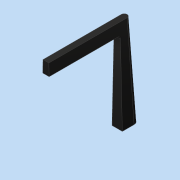
# Autodesk Inventor part: RudderStabilizingFins
Saved by Autodesk Inventor 2017 (Build 210142000, 142)
## iProperties
Created: 2016-10-10
Part Number: RudderStabilizingFins
Material: Generic
Document SubType Name: Modeling
Designer: techn
Density: 1 g/cm^3
Appearance: Glossy - Black
Author: techn
Autodesk Inventor part; units mm, degrees
ref_plane "YZ Plane" through (0, 0, 0) normal (1, 0, 0) x (0, 1, 0)
ref_plane "XY Plane" through (0, 0, 0) normal (0, 0, 1) x (1, 0, 0)
sketch "Sketch6" plane through (0, 0, 0) normal (0, 1, 0) x (-1, 0, 0)
  line L0 (0, 0) -> (5.588, 0)
  line L1 (5.588, 0) -> (5.588, -6.35)
  line L2 (5.588, -6.35) -> (0, -6.35)
  line L3 (0, -6.35) -> (0, 0)
  arc A0 (0, -6.35) -> (5.588, -6.35) centre (2.794, -6.35) ccw
  dimension "d25" = 5.588
  dimension "d26" = 6.35
  constraints: 8 end point, 2 parallel, 2 point on circle, 2 tangent, 1 centre point, 1 horizontal, 1 perpendicular
  measures "d25" distance of L1.end L2.end
  measures "d26" distance of L0.end L1.end
ref_plane "Work Plane1" through (0, 50.8, 0) normal (0, 1, 0) x (-1, 0, 0)
sketch "Sketch8" plane through (0, 50.8, 0) normal (0, 1, 0) x (-1, 0, 0)
  line L0 (4.3815, 0) -> (1.2065, 0)
  line L1 (1.2065, 0) -> (1.2065, -3.81)
  line L2 (1.2065, -3.81) -> (4.3815, -3.81)
  line L3 (4.3815, -3.81) -> (4.3815, 0)
  arc A0 (1.2065, -3.81) -> (4.3815, -3.81) centre (2.794, -3.81) ccw
  point P0 (0, 0)
  dimension "d27" = 3.175
  dimension "d28" = 3.81
  dimension "d49" = 1.2065
  constraints: 8 end point, 2 parallel, 2 point on circle, 2 tangent, 1 centre point, 1 horizontal, 1 perpendicular, 1 point on line
  measures "d27" distance of L2.end L1.end
  measures "d28" distance of L1.end L0.end
  measures "d49" distance from line of point (0, 0) L1
loft "Loft1" add profiles "Sketch6", "Sketch8"
sketch "Sketch9" plane through (-5.588, 0, 0) normal (0, 0, 1) x (1, 0, 0)
  line L0 (0, 0) -> (5.588, 0) projected
  line L1 (5.588, 0) -> (4.3815, 50.8) projected
  line L2 (1.2065, 50.8) -> (4.3815, 50.8) projected
  line L3 (0, 0) -> (1.2065, 50.8) projected
  line L4 (4.3815, 50.8) -> (5.588, 0) projected
  line L5 (4.5323, 44.45) -> (1.0557, 44.45)
  line L6 (0, 0) -> (1.2065, 50.8) projected
  dimension "d34" = 6.35
  constraints: 2 end point, 2 point on line, 1 horizontal
  measures "d34" distance between parallel lines of L2 L5
extrude "Extrusion5" add sketch "Sketch9" along normal blind 38.608 contours L3 L2 L1 L5
fillet "Fillet2" radius 1.5875 1 edges at (-2.794, 44.45, 0)
sketch "Sketch12" plane through (-2.794, 0, -6.35) normal (0, -1, 0) x (1, 0, 0)
  circle A0 centre (0, 1.9685) radius 1.27
  arc A1 (-2.794, 0) -> (2.794, 0) centre (0, 0) ccw projected
  line L0 (0, -2.794) -> (0, 1.9685)
  point P0 (2.794, 6.35)
  dimension "d44" = 2.54
  dimension "d46" = 4.7625
  constraints: 2 end point, 1 centre point, 1 point on circle, 1 vertical
  measures "d44" diameter of A0
  measures "d46" distance of L0.start L0.end
extrude "Extrusion8" cut sketch "Sketch12" against normal blind 10.16
body "Solid4"
